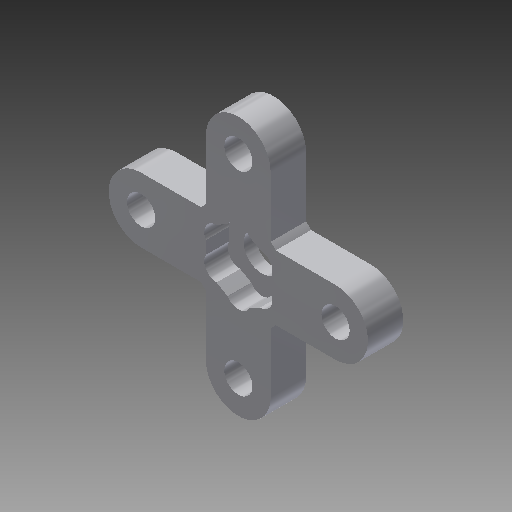
# Autodesk Inventor part: 付け根_フリー軸
Saved by Autodesk Inventor 2018 (Build 220112000, 112)
## iProperties
Category: 付け根
Created: 2016-05-01
Part Number: 付け根_フリー軸
Material: アルミニウム 2014-T4
Document SubType Name: Modeling
Designer: hiroaki
Density: 2.8 g/cm^3
Appearance: サテン
Mass: 1.34572 g
Surface Area: 7.19277 cm^2
Volume: 0.480616 cm^3
Author: hiroaki
Autodesk Inventor part; units mm, degrees
ref_plane "YZ Plane" through (0, 0, 0) normal (1, 0, 0) x (0, 1, 0)
ref_plane "XZ Plane" through (0, 0, 0) normal (0, 1, 0) x (-1, 0, 0)
ref_plane "XY Plane" through (0, 0, 0) normal (0, 0, 1) x (1, 0, 0)
sketch "スケッチ1" plane through (0, 0, 0) normal (0, 0, 1) x (1, 0, 0)
  circle A0 centre (0, 0) radius 1.55
  circle A1 centre (0, 0) radius 2.5 construction
  circle A2 centre (0, 8.25) radius 1.2
  circle A3 centre (0, 8.25) radius 2.75 construction
  circle A4 centre (0, 8.25) radius 3.75 construction
  circle A5 centre (-8.25, 0) radius 1.2
  circle A6 centre (0, -8.25) radius 1.2
  circle A7 centre (8.25, 0) radius 1.2
  circle A8 centre (0, 0) radius 5.5 construction
  arc A9 (2.75, 8.25) -> (-2.75, 8.25) centre (0, 8.25) ccw
  line L0 (-2.75, 8.25) -> (-2.75, 3.1745)
  line L1 (-8.25, 2.75) -> (-3.1745, 2.75)
  arc A10 (-8.25, 2.75) -> (-8.25, -2.75) centre (-8.25, 0) ccw
  line L2 (-8.25, -2.75) -> (-3.1745, -2.75)
  line L3 (-2.75, -3.1745) -> (-2.75, -8.25)
  line L4 (2.75, 8.25) -> (2.75, 3.1745)
  line L5 (3.1745, 2.75) -> (8.25, 2.75)
  line L6 (8.25, -2.75) -> (3.1745, -2.75)
  line L7 (2.75, -3.1745) -> (2.75, -8.25)
  arc A11 (8.25, -2.75) -> (8.25, 2.75) centre (8.25, 0) ccw
  arc A12 (-2.75, -8.25) -> (2.75, -8.25) centre (0, -8.25) ccw
  circle A13 centre (0, 0) radius 3.2 construction
  arc A14 (-2.75, 3.1745) -> (-3.1745, 2.75) centre (0, 0) ccw
  arc A15 (-3.1745, -2.75) -> (-2.75, -3.1745) centre (0, 0) ccw
  arc A16 (3.1745, 2.75) -> (2.75, 3.1745) centre (0, 0) ccw
  arc A17 (2.75, -3.1745) -> (3.1745, -2.75) centre (0, 0) ccw
  dimension "d0" = 3.1
  dimension "d1" = 5
  dimension "d2" = 2.4
  dimension "d3" = 5.5
  dimension "d4" = 1
  dimension "d7" = 360
  dimension "d22" = 11
  dimension "d24" = 6.4
  dimension "d25" = 1
  constraints: 18 centre point, 16 end point, 16 point on circle, 14 coincident, 10 tangent, 6 equal radius, 3 horizontal, 3 perpendicular, 2 vertical, 1 vertical alignment, 9 other
  measures "d0" diameter of A0
  measures "d1" diameter of A1
  measures "d2" diameter of A2
  measures "d3" diameter of A3
  measures "d4" radial gap between concentric circles of A3 A4
  measures "d22" diameter of A8
  measures "d24" diameter of A13
  measures "d25" radial gap between concentric circles of A13 A14
extrude "押し出し1" add sketch "スケッチ1" along normal blind 3
sketch "スケッチ6" plane through (0, 0, 3) normal (0, 0, 1) x (1, 0, 0)
  circle A0 centre (0, 0) radius 1.55 projected
  arc A1 (3.1745, 2.75) -> (2.75, 3.1745) centre (0, 0) ccw projected
  line L0 (-2.75, -1.5877) -> (-2.75, 1.5877)
  line L1 (-2.75, 1.5877) -> (0, 3.1754)
  line L2 (0, 3.1754) -> (2.75, 1.5877)
  line L3 (2.75, 1.5877) -> (2.75, -1.5877)
  line L4 (2.75, -1.5877) -> (0, -3.1754)
  line L5 (0, -3.1754) -> (-2.75, -1.5877)
  line L6 (0, -3.1812) -> (2.755, -1.5906)
  line L7 (2.755, -1.5906) -> (2.755, 1.5906)
  line L8 (2.755, 1.5906) -> (0, 3.1812)
  line L9 (0, 3.1812) -> (-2.755, 1.5906)
  line L10 (-2.755, 1.5906) -> (-2.755, -1.5906)
  line L11 (-2.755, -1.5906) -> (0, -3.1812)
  circle A2 centre (0, -2.1312) radius 1.05
  circle A3 centre (1.8457, -1.0656) radius 1.05
  circle A4 centre (1.8457, 1.0656) radius 1.05
  circle A5 centre (0, 2.1312) radius 1.05
  circle A6 centre (-1.8457, 1.0656) radius 1.05
  circle A7 centre (-1.8457, -1.0656) radius 1.05
  point P0 (2.755, -1.5906)
  point P1 (2.755, 1.5906)
  point P2 (0, 3.1812)
  point P3 (-2.755, 1.5906)
  point P4 (-2.755, -1.5906)
  dimension "d28" = 2.1
  dimension "d26" = 5.5
  dimension "d27" = 0.005
  dimension "d31" = 360
  constraints: 24 end point, 3 vertical alignment, 1 coincident, 1 vertical, 53 other
  measures "d26" distance between parallel lines of L0 L3
  measures "d27" distance between parallel lines of L6 L4
extrude "押し出し3" cut sketch "スケッチ6" against normal blind 2 contours A0 A4 L3 A3 | A4 A0 | A4 L8 | A0 A4 L2 L3 | A3 L7 L6 A0 | A0 A3 | A0 A5 L2 A4 | L3 L2 L8 L7 | L7 A4 | A3 L4 A2 A0 | A3 L7 | A5 A0 | A0 A5 L1 L2 | A2 L4 L5 A0 | A0 A2 | L6 A3 | A0 A6 L1 A5 | L2 L1 L9 L8 | L8 A5 | A2 L5 A7 A0 | L6 L11 L5 L4 | A2 L6 | A6 A0 | A0 A6 L10 L9 | A5 L9 | A7 L11 | A7 L5 L0 A0 | A0 A7 | L11 A2 | A0 A7 L0 A6 | L9 A6 | L10 A7 | L11 L10 L0 L5 | A6 L10
